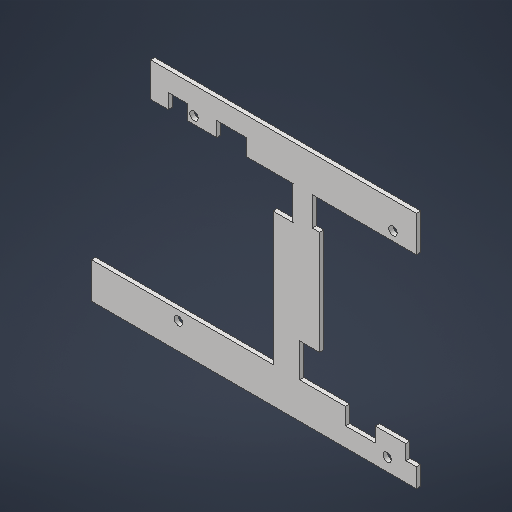
# Autodesk Inventor part: PCB_interface_v2
Saved by Autodesk Inventor 2027.1 (Build 311270010, 270A)
## iProperties
Created: 2026-09-14
Part Number: PCB_interface_v2
Material: Generic
Document SubType Name: Modeling
Designer: szymo
Density: 1 g/cm^3
Appearance: Default
Author: szymo
Autodesk Inventor part; units mm, degrees
ref_plane "YZ Plane" through (0, 0, 0) normal (1, 0, 0) x (0, 1, 0)
ref_plane "XZ Plane" through (0, 0, 0) normal (0, 1, 0) x (-1, 0, 0)
ref_plane "XY Plane" through (0, 0, 0) normal (0, 0, 1) x (1, 0, 0)
sketch "Sketch1" plane through (0, 0, 0) normal (0, 0, 1) x (1, 0, 0)
  circle A0 centre (-5.7295, 41.15) radius 1.0065 projected
  circle A1 centre (-52.875, 41.15) radius 1.0065 projected
  line L0 (-57.9354, 38.4) -> (-57.9354, 42.4) projected
  line L1 (-57.9354, 42.4) -> (-55.625, 42.4) projected
  line L2 (-55.625, 42.4) -> (-55.625, 38.4) projected
  line L3 (-55.625, 38.4) -> (-46.3947, 38.4) projected
  line L4 (-46.3947, 38.4) -> (-46.3947, 42.4) projected
  line L5 (-46.3947, 42.4) -> (-41.4006, 42.4) projected
  line L6 (-41.4006, 42.4) -> (-41.4006, 38.4) projected
  line L7 (-41.4006, 38.4) -> (0, 38.4) projected
  line L8 (0, 38.4) -> (0, 47.7) projected
  line L9 (0, 47.7) -> (-59.3371, 47.7) projected
  line L10 (-59.3371, 38.4) -> (-59.3371, 47.7) projected
  line L11 (-59.3371, 38.4) -> (-57.9354, 38.4) projected
  circle A2 centre (-56.5871, -2.75) radius 1.0065 projected
  circle A3 centre (-7.1235, -6) radius 1.0065 projected
  line L12 (-15.9365, -4) -> (-15.9365, 0) projected
  line L13 (-59.3371, 0) -> (-15.9365, 0) projected
  line L14 (-59.3371, 0) -> (-59.3371, -9.3) projected
  line L15 (-59.3371, -9.3) -> (0, -9.3) projected
  line L16 (0, -4) -> (0, -9.3) projected
  line L17 (0, -4) -> (-1.712, -4) projected
  line L18 (-1.712, -4) -> (-1.712, 0) projected
  line L19 (-10.9424, 0) -> (-1.712, 0) projected
  line L20 (-10.9424, 0) -> (-10.9424, -4) projected
  line L21 (-10.9424, -4) -> (-15.9365, -4) projected
  line L22 (-77.2, -9) -> (-65.2, -9)
  line L23 (-65.2, -9) -> (-65.2, 11)
  line L24 (-65.2, 11) -> (-77.2, 11)
  line L25 (-77.2, 11) -> (-77.2, -9)
  line L26 (-77.2, -9) -> (-0.2, -9)
  line L27 (-0.2, -9) -> (-0.2, -4.5)
  line L28 (-0.2, -4.5) -> (-2.7272, -4.5)
  line L29 (-2.7272, -4.5) -> (-2.7272, -1)
  line L30 (-2.7272, -1) -> (-9.9272, -1)
  line L31 (-9.9272, -1) -> (-9.9272, -4.5)
  line L32 (-9.9272, -4.5) -> (-17, -4.5)
  line L33 (-17, -4.5) -> (-17, -0.5)
  line L34 (-17, -0.5) -> (-77.2, -0.5)
  line L35 (-61.3371, -12.3) -> (-59.4157, -12.3) projected
  line L36 (-59.4157, -12.3) -> (-59.3371, -12.3) projected
  line L37 (-59.3371, 0) -> (-59.3371, -12.3) projected
  line L38 (-59.3371, 0) -> (-63.3371, 0) projected
  line L39 (-63.3371, 0) -> (-63.3371, -6.8) projected
  line L40 (-63.3371, -6.8) -> (-63.3371, -14.3) projected
  arc A4 (-61.3371, -12.3) -> (-63.3371, -14.3) centre (-61.3371, -14.3) ccw projected
  line L41 (-59.3371, 50.7) -> (-59.4157, 50.7) projected
  line L42 (-59.4157, 50.7) -> (-61.3371, 50.7) projected
  arc A5 (-63.3371, 52.7) -> (-61.3371, 50.7) centre (-61.3371, 52.7) ccw projected
  line L43 (-63.3371, 44.7) -> (-63.3371, 52.7) projected
  line L44 (-63.3371, 38.4) -> (-63.3371, 44.7) projected
  line L45 (-63.3371, 38.4) -> (-59.3371, 38.4) projected
  line L46 (-59.3371, 38.4) -> (-59.3371, 50.7) projected
  line L47 (-63.2, 47.5) -> (-0.2, 47.5)
  line L48 (-0.2, 47.5) -> (-0.2, 39)
  line L49 (-63.2, 39.4) -> (-63.2, 47.5)
  line L50 (6.5, 33.15) -> (-22.9, 33.15) projected
  line L51 (-34.4371, 33.15) -> (-63.8371, 33.15) projected
  line L52 (-34.4371, 5.25) -> (-63.8371, 5.25) projected
  line L53 (6.5, 5.25) -> (-22.9, 5.25) projected
  line L54 (-0.2, 39) -> (-40.4, 39)
  line L55 (-40.4, 39) -> (-40.4, 42.9)
  line L56 (-40.4, 42.9) -> (-47.5099, 42.9)
  line L57 (-47.5099, 42.9) -> (-47.5099, 39.4)
  line L58 (-47.5099, 39.4) -> (-54.5099, 39.4)
  line L59 (-54.5099, 39.4) -> (-54.5099, 42.9)
  line L60 (-54.5099, 42.9) -> (-59, 42.9)
  line L61 (-59, 42.9) -> (-59, 39.4)
  line L62 (-59, 39.4) -> (-63.2, 39.4)
  line L63 (-27.9, -0.5) -> (-27.9, 7.5)
  line L64 (-27.9, 7.5) -> (-23.1685, 7.5)
  line L65 (-23.1685, 7.5) -> (-23.1685, 32.15)
  line L66 (-23.1685, 32.15) -> (-24.9, 32.15)
  line L67 (-24.9, 32.15) -> (-24.9, 39)
  line L68 (-29.4371, 39) -> (-29.4371, 31)
  line L69 (-29.4371, 31) -> (-34.1685, 31)
  line L70 (-34.1685, 31) -> (-34.1685, -0.5)
  point P0 (0, 0)
  point P1 (-24.9, 38.4)
  point P2 (-29.4371, 38.4)
  dimension "d0" = 12
  dimension "d1" = 20
  dimension "d3" = 0.3
  dimension "d4" = 8.5
  dimension "d5" = 0.5
  dimension "d6" = 4.5
  dimension "d7" = 0.5
  dimension "d8" = 8
  dimension "d9" = 1
  dimension "d10" = 7.2
  dimension "d11" = 1.0152
  dimension "d12" = 1.0152
  dimension "d14" = 0.2
  dimension "d15" = 77
  dimension "d16" = 60.2
  dimension "d17" = 1.0635
  dimension "d18" = 0.2
  dimension "d19" = 0.2
  dimension "d21" = 63
  dimension "d23" = 8.5
  dimension "d24" = 1
  dimension "d25" = 0.5
  dimension "d27" = 4.2
  dimension "d28" = 1.0646
  dimension "d29" = 1.1152
  dimension "d30" = 1.1152
  dimension "d31" = 7
  dimension "d32" = 8.1
  dimension "d33" = 1.0006
  dimension "d34" = 40.2
  dimension "d35" = 8
  dimension "d36" = 8
  dimension "d38" = 0.2685
  dimension "d39" = 0.2685
  dimension "d40" = 11
  dimension "d41" = 5
  dimension "d42" = 5
  dimension "d43" = 1
  dimension "d44" = 2
  constraints: 66 end point, 20 perpendicular, 9 point on line, 5 horizontal, 3 parallel, 3 vertical
  measures "d0" distance of L24.end L23.end
  measures "d1" distance of L23.end L22.end
  measures "d3" distance between parallel lines of L26 L15
  measures "d4" distance between parallel lines of L34 L26
  measures "d5" distance between parallel lines of L13 L34
  measures "d6" distance between parallel lines of L26 L32
  measures "d7" distance between parallel lines of L21 L32
  measures "d8" distance between parallel lines of L26 L30
  measures "d9" distance between parallel lines of L19 L30
  measures "d10" distance between parallel lines of L31 L29
  measures "d11" distance between parallel lines of L18 L29
  measures "d12" distance between parallel lines of L20 L31
  measures "d14" distance between parallel lines of L16 L27
  measures "d15" distance between parallel lines of L25 L27
  measures "d16" distance between parallel lines of L33 L25
  measures "d17" distance between parallel lines of L12 L33
  measures "d18" distance between parallel lines of L8 L48
  measures "d19" distance between parallel lines of L9 L47
  measures "d21" distance between parallel lines of L48 L49
  measures "d23" distance between parallel lines of L47 L54
  measures "d24" distance between parallel lines of L3 L58
  measures "d25" distance between parallel lines of L60 L1
  measures "d27" distance between parallel lines of L49 L61
  measures "d28" distance between parallel lines of L0 L61
  measures "d29" distance between parallel lines of L59 L2
  measures "d30" distance between parallel lines of L4 L57
  measures "d31" distance between parallel lines of L57 L59
  measures "d32" distance between parallel lines of L47 L58
  measures "d33" distance between parallel lines of L6 L55
  measures "d34" distance between parallel lines of L48 L55
  measures "d35" distance between parallel lines of L64 L34
  measures "d36" distance between parallel lines of L54 L69
  measures "d38" distance from line of L65 L50.end
  measures "d39" distance from line of L70 L51.start
  measures "d40" distance between parallel lines of L65 L70
  measures "d41" distance from line of L53.end L63
  measures "d42" distance from line of L51.start L68
  measures "d43" distance from line of L66 L50.end
  measures "d44" distance from line of L50.end L67
extrude "Extrusion1" add sketch "Sketch1" along normal blind 1 contours L62 L49 L47 L10 | L10 L47 L48 L54 L55 L56 L57 L58 L59 L60 L61 L62 | L67 L7 L68 L54 | L67 L66 L65 L64 L63 L13 L70 L69 L68 L7 | L13 L63 L34 L70 | L34 L33 L32 L31 L30 L29 L28 L27 L26 L14 | L14 L26 L40 L39 L34 | L39 L40 L26 L23 L34 | L23 L22 L25 L34
equation "\"d11\" = d12"
equation "\"d23\" = d4"
equation "\"d25\" = d7"
equation "\"d30\" = d29"
equation "\"d36\" = d35"
equation "\"d39\" = d38"
equation "\"d42\" = d41"
body "Solid1"
